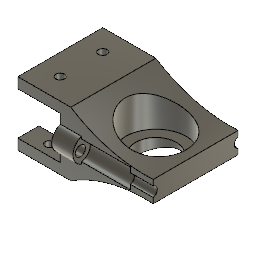
Chassis_Design v17 (Autodesk Fusion 360 archive; units mm, degrees)
design "upperBracket_vFINAL"
Autodesk Fusion 360 part; units mm, degrees
sketch "Sketch1" plane through (0, 0, 0) normal (0, 1, 0) x (1, 0, 0)
  line L0 (0, 0) -> (0, -10)
  line L1 (0, -10) -> (-20, -10)
  line L2 (-20, -10) -> (-20, -15)
  line L3 (-20, -15) -> (5, -15)
  arc A0 (43.7298, -5) -> (5, -15) centre (39.8266, -69.8827) ccw
  line L4 (43.7298, -5) -> (43.7298, 0)
  line L5 (0, 0) -> (43.7298, 0)
  line L6 (0, 10) -> (-20, 10)
  line L7 (-20, 15) -> (5, 15)
  line L8 (0, 0) -> (0, 10)
  arc A1 (5, 15) -> (43.7298, 5) centre (39.8266, 69.8827) ccw
  line L9 (43.7298, 5) -> (43.7298, 0)
  line L10 (-20, 10) -> (-20, 15)
  dimension "d2" = 10
  dimension "d3" = 5
  dimension "d4" = 25
  dimension "d5" = 5
  dimension "d6" = 65
  dimension "d11" = 40
  constraint coincident L0.start L5.start
  constraint vertical L0
  constraint perpendicular L0 L1
  constraint perpendicular L1 L2
  constraint perpendicular L2 L3
  constraint vertical L4
  constraint perpendicular L4 L5
  constraint symmetric L0.start L5 L8.start
  constraint symmetric L0.end L5 L6.start
  constraint symmetric L1.end L5 L6.end
  constraint symmetric L2.end L5 L7.start
  constraint symmetric L3.end L5 L7.end
  constraint symmetric A0.start L5 A1.end
  constraint symmetric A0 L5 A1
  constraint symmetric L4.end L5 L9.end
  measures "d2" distance of L0.start L0.end
  measures "d3" distance of L1.end L2.end
  measures "d4" distance of L2.end L3.end
  measures "d5" distance of A0.start L4.end
  measures "d6" radius of A0
  measures "d11" distance of L3.end A0.start
extrude "Extrude1" add sketch "Sketch1" along normal mid plane 40
sketch "Sketch2" plane through (0, 0, 0) normal (0, 0, 1) x (1, 0, 0)
  circle A0 centre (25, 0) radius 14.2875
  dimension "d10" = 28.575
  dimension "d56" = 25
  measures "d10" diameter of A0
  measures "d56" distance of origin A0.centre
extrude "Extrude2" cut sketch "Sketch2" along normal blind 20 and the other way blind 4
sketch "Sketch3" plane through (0, 0, 15) normal (0, 0, 1) x (-1, 0, 0)
  line L0 (-5, 20) -> (-5, -20)
  line L1 (-5, -20) -> (20, -20)
  line L2 (20, -20) -> (20, 20)
  line L3 (20, 20) -> (-5, 20)
  circle A0 centre (10, -10) radius 2
  circle A1 centre (10, 10) radius 2
  dimension "d14" = 4
  dimension "d15" = 4
  dimension "d16" = 10
  dimension "d17" = 10
  dimension "d18" = 10
  dimension "d19" = 10
  measures "d14" diameter of A0
  measures "d15" diameter of A1
  measures "d16" distance of L2 A0.centre
  measures "d17" distance of L2 A1.centre
  measures "d18" distance of L1 A0.centre
  measures "d19" distance of L3 A1.centre
extrude "Extrude3" cut sketch "Sketch3" against normal up to surface (5 mm away) contours A0 | A1
sketch "Sketch7" plane through (0, 0, -15) normal (0, 0, -1) x (1, 0, 0)
  line L0 (-20, 20) -> (-20, -20)
  line L1 (-20, -20) -> (5, -20)
  line L2 (5, -20) -> (5, 20)
  line L3 (5, 20) -> (-20, 20)
  line L4 (-20, 0) -> (-20, -10)
  line L5 (-20, -10) -> (0, -10)
  line L6 (0, -10) -> (0, 10)
  line L7 (0, 10) -> (-20, 10)
  line L8 (-20, 10) -> (-20, 0)
  constraint vertical L4
  constraint perpendicular L2 L5
  constraint perpendicular L5 L6
  constraint coincident L0 L7.end
  constraint perpendicular L0 L7
  constraint perpendicular L7 L8
extrude "Extrude6" cut sketch "Sketch7" against normal blind 10 contours L0 L4 L5 L6 L7 L8
sketch "Sketch8" plane through (0, 0, -10) normal (0, 0, 1) x (-1, 0, 0)
  line L0 (20, -10) -> (0, -10)
  line L1 (0, -10) -> (0, -20)
  line L2 (0, -20) -> (20, -20)
  line L3 (20, -20) -> (20, -10)
  circle A0 centre (10, -15) radius 2
  circle A1 centre (10, 15) radius 2
  line L4 (20, 20) -> (20, 10)
  line L5 (0, 10) -> (20, 10)
  dimension "d36" = 4
  dimension "d37" = 10
  dimension "d38" = 5
  dimension "d39" = 4
  dimension "d40" = 10
  dimension "d41" = 5
  measures "d36" diameter of A0
  measures "d37" distance of L3 A0.centre
  measures "d38" distance of L0 A0.centre
  measures "d39" diameter of A1
  measures "d40" distance of A1.centre L4
  measures "d41" distance of A1.centre L5
extrude "Extrude7" cut sketch "Sketch8" against normal up to surface (5 mm away) contours A0 | A1
sketch "Sketch9" plane through (0, 0, 0) normal (-1, 0, 0) x (0, -1, 0)
  line L0 (10, -10) -> (20, -10)
  line L1 (-10, -10) -> (-10, -15)
  line L2 (-10, -15) -> (10, -15)
  line L3 (10, -15) -> (10, -10)
  line L4 (20, 10) -> (-20, 10)
  circle A0 centre (-18, 0) radius 6
  circle A1 centre (18, 0) radius 6
  line L5 (20, -10) -> (20, 10)
  line L6 (-20, 10) -> (-20, -10)
  line L7 (-20, -10) -> (-10, -10)
  dimension "d46" = 12
  dimension "d47" = 12
  measures "d46" diameter of A0
  measures "d47" diameter of A1
extrude "Extrude8" add sketch "Sketch9" against normal blind 10 contours A1 L5 | A0 L6 picked at (21.1814, -1.7134) picked at (-21.347, -0.8549)
sketch "Sketch10" plane through (0, 0, 0) normal (-1, 0, 0) x (0, -1, 0)
  line L0 (10, -10) -> (20, -10)
  line L1 (-10, -10) -> (-10, -15)
  line L2 (-10, -15) -> (10, -15)
  line L3 (10, -15) -> (10, -10)
  arc A0 (20, -5.6569) -> (20, 5.6569) centre (18, 0) ccw
  line L4 (20, 10) -> (-20, 10)
  arc A1 (-20, 5.6569) -> (-20, -5.6569) centre (-18, 0) ccw
  circle A2 centre (-20.5, 0) radius 2.4
  circle A3 centre (20.5, 0) radius 2.4
  line L5 (20, -10) -> (20, -5.6569)
  line L6 (20, 5.6569) -> (20, 10)
  line L7 (-20, 10) -> (-20, 5.6569)
  line L8 (-20, -5.6569) -> (-20, -10)
  line L9 (-20, -10) -> (-10, -10)
  dimension "d50" = 4.8
  dimension "d51" = 2.5
  dimension "d52" = 2.5
  dimension "d53" = 4.8
  measures "d50" diameter of A2
  measures "d51" distance of A1.centre A2.centre
  measures "d52" distance of A0.centre A3.centre
  measures "d53" diameter of A3
extrude "Extrude9" cut sketch "Sketch10" against normal up to surface (43.7298 mm away) contours A2 | A3
sketch "Sketch11" plane through (0, 0, -4) normal (0, 0, 1) x (-1, 0, 0)
  circle A0 centre (-25, 0) radius 14.2875
  circle A1 centre (-25, 0) radius 9.525
  dimension "d59" = 19.05
  constraint concentric A0 A1
  measures "d59" diameter of A1
extrude "Extrude10" cut sketch "Sketch11" along normal up to surface contours A1 end surface at (7.3183, 6.6667, -13.5958)
sketch "Sketch12" plane through (10, 0, 0) normal (1, 0, 0) x (0, 1, 0)
  arc A0 (20, -2.3473) -> (20, 2.3473) centre (20.5, 0) ccw
  line L0 (20, -2.3473) -> (20, -5.6569)
  arc A1 (20, -5.6569) -> (20, 5.6569) centre (18, 0) ccw
  line L1 (20, 5.6569) -> (20, 2.3473)
  circle A2 centre (-20.5, 0) radius 4.65
  arc A3 (-20, 2.3473) -> (-20, -2.3473) centre (-20.5, 0) ccw
  circle A4 centre (20.5, 0) radius 4.65
  dimension "d62" = 9.3
  dimension "d63" = 9.3
  constraint concentric A2 A3
  constraint concentric A0 A4
  measures "d62" diameter of A2
  measures "d63" diameter of A4
extrude "Extrude11" cut sketch "Sketch12" along normal blind 23 contours A0 L0 L1 A4 | A2
equation "d39 = d36"
equation "d40 = d37"
equation "d41 = d38"
equation "d47 = d46"
equation "d52 = d51"
equation "d53 = d50"
